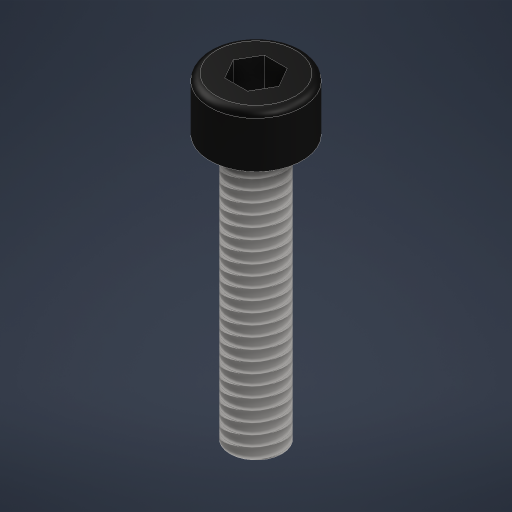
# Autodesk Inventor part: M4x20
Saved by Autodesk Inventor 2024 (Build 280153000, 153)
## iProperties
Created: 2024-10-26
Part Number: M4x20
Material: Generic
Document SubType Name: Modeling
Designer: jerem
Density: 1 g/cm^3
Appearance: Default
Author: jerem
Autodesk Inventor part; units mm, degrees
ref_plane "YZ Plane" through (0, 0, 0) normal (1, 0, 0) x (0, 1, 0)
ref_plane "XZ Plane" through (0, 0, 0) normal (0, 1, 0) x (-1, 0, 0)
ref_plane "XY Plane" through (0, 0, 0) normal (0, 0, 1) x (1, 0, 0)
sketch "Sketch1" plane through (0, 0, 0) normal (0, 1, 0) x (-1, 0, 0)
  circle A0 centre (0, 0) radius 1.97
  circle A1 centre (0, 0) radius 3.5
  line L0 (0.866, -1.5) -> (-0.866, -1.5)
  line L1 (-0.866, -1.5) -> (-1.7321, 0)
  line L2 (-1.7321, 0) -> (-0.866, 1.5)
  line L3 (-0.866, 1.5) -> (0.866, 1.5)
  line L4 (0.866, 1.5) -> (1.7321, 0)
  line L5 (1.7321, 0) -> (0.866, -1.5)
  dimension "d0" = 3.94
  dimension "d1" = 7
  dimension "d8" = 3
  constraints: 12 end point, 3 coincident, 2 centre point, 1 horizontal, 13 other
  measures "d0" diameter of A0
  measures "d1" diameter of A1
  measures "d8" distance between parallel lines of L3 L0
extrude "Extrusion1" add sketch "Sketch1" along normal blind 4 contours A0 | A1 | L0 L1 L2 L3 L4 L5
extrude "Extrusion2" add sketch "Sketch1" against normal blind 20 contours A0 | L0 L1 L2 L3 L4 L5
extrude "Extrusion3" cut sketch "Sketch1" against normal blind 3 from surface at 4 contours L0 L1 L2 L3 L4 L5
fillet "Fillet1" radius 0.5 1 edges at (3.5, 4, 0)
thread "Thread2" size "M5x0.8" class "6g" standard "ANSI Metric M Profile" full length
equation "\"d4\" = length"
equation "\"length\" = 20"
body "Solid1"
